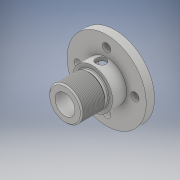
# Autodesk Inventor part: РК3
Saved by Autodesk Inventor 2019.3 (Build 233278000, 278)
## iProperties
Created: 2020-04-01
Part Number: РК3
Material: Типовые
Document SubType Name: Modeling
Designer: Admin
Density: 1 g/cm^3
Appearance: По умолчанию
Mass: 94.6914 g
Surface Area: 289.936 cm^2
Volume: 94.6914 cm^3
Author: Admin
Autodesk Inventor part; units mm, degrees
ref_plane "YZ Plane" through (0, 0, 0) normal (1, 0, 0) x (0, 1, 0)
ref_plane "XZ Plane" through (0, 0, 0) normal (0, 1, 0) x (-1, 0, 0)
ref_plane "XY Plane" through (0, 0, 0) normal (0, 0, 1) x (1, 0, 0)
sketch "Эскиз1" plane through (0, 0, 0) normal (0, 0, 1) x (1, 0, 0)
  circle A0 centre (0, 0) radius 47.5
  dimension "d0" = 95
  constraints: 1 centre point, 1 coincident
  measures "d0" diameter of A0
extrude "Выдавливание1" add sketch "Эскиз1" along normal blind 10
sketch "Эскиз2" plane through (0, 0, 10) normal (0, 0, 1) x (1, 0, 0)
  circle A0 centre (0, 0) radius 24
  dimension "d3" = 48
  constraints: 1 centre point, 1 coincident
  measures "d3" diameter of A0
extrude "Выдавливание2" add sketch "Эскиз2" along normal blind 17
sketch "Эскиз4" plane through (0, 0, 10) normal (0, 0, 1) x (1, 0, 0)
  line L0 (0, 0) -> (34, 0)
  circle A0 centre (34, 0) radius 5
  circle A1 centre (0, 34) radius 5
  circle A2 centre (-34, 0) radius 5
  circle A3 centre (0, -34) radius 5
  dimension "d9" = 34
  dimension "d10" = 10
  dimension "d13" = 360
  constraints: 4 centre point, 2 end point, 1 coincident, 1 horizontal, 9 other
  measures "d9" distance of L0.start L0.end
  measures "d10" diameter of A0
extrude "Выдавливание4" cut sketch "Эскиз4" against normal through all
sketch "Эскиз5" plane through (0, 0, 0) normal (0, 1, 0) x (-1, 0, 0)
  line L0 (0, 27) -> (0, 60)
  line L1 (0, 60) -> (20, 60)
  line L2 (20, 60) -> (20, 32.3071)
  line L3 (20, 32.3071) -> (19.0464, 31.3536)
  line L4 (18.9, 31) -> (18.9, 28)
  arc A0 (18.9, 28) -> (19.9, 27) centre (19.9, 28) ccw
  arc A1 (19.0464, 31.3536) -> (18.9, 31) centre (19.4, 31) ccw
  line L5 (0, 27) -> (19.9, 27)
  line L6 (24, 27) -> (-24, 27) projected
  line L7 (0, -12) -> (0, 72) projected
  point P0 (0, 0)
  dimension "d17" = 33
  dimension "d18" = 20
  dimension "d19" = 18.9
  dimension "d20" = 1
  dimension "d21" = 45
  dimension "d22" = 0.5
  constraints: 12 end point, 4 point on circle, 4 tangent, 2 centre point, 2 vertical, 1 collinear, 1 perpendicular
  measures "d17" distance of L0.start L0.end
  measures "d18" distance of L0.end L1.end
  measures "d19" distance between parallel lines of L0 L4
  measures "d20" radius of A0
  measures "d21" angle of L2 L3
  measures "d22" radius of A1
revolve "Вращение1" add sketch "Эскиз5" angle 360 about axis through (0, 0, -10) along (0, 0, 1)
chamfer "Фаска1" distance 1.6 angle 45 1 edges at (20, 0, 60)
thread "Резьба1" size "M40x1.5" class "6g" standard "ANSI Metric M Profile" full length
sketch "Эскиз6" plane through (0, 0, 60) normal (0, 0, 1) x (1, 0, 0)
  circle A0 centre (0, 0) radius 12
  dimension "d30" = 24
  constraints: 1 centre point, 1 coincident
  measures "d30" diameter of A0
sketch "Эскиз7" plane through (0, 0, 0) normal (0, 0, -1) x (-1, 0, 0)
  circle A0 centre (0, 0) radius 20
  dimension "d31" = 40
  constraints: 1 centre point, 1 coincident
  measures "d31" diameter of A0
extrude "Выдавливание5" cut sketch "Эскиз7" against normal blind 20
extrude "Выдавливание6" cut sketch "Эскиз6" against normal through all
sketch "Эскиз8" plane through (0, 0, 0) normal (0, 1, 0) x (-1, 0, 0)
  circle A0 centre (0, 17) radius 6
  line L0 (0, -16.4988) -> (0, 98.9927) projected
  line L1 (47.5, 10) -> (-47.5, 10) projected
  point P0 (0, 0)
  dimension "d36" = 12
  dimension "d37" = 7
  constraints: 1 centre point, 1 point on line
  measures "d36" diameter of A0
  measures "d37" distance from line of A0.centre L1
extrude "Выдавливание7" cut sketch "Эскиз8" along normal through all both and the other way through all
